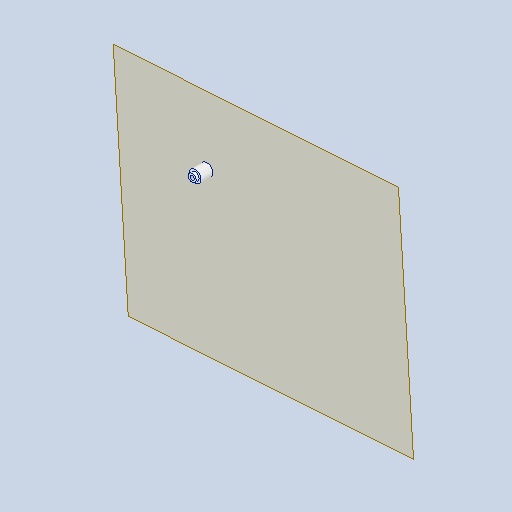
# Autodesk Inventor part: návarek na stěnu
Saved by Autodesk Inventor 2023 (Build 270158000, 158)
## iProperties
Created: 2023-04-03
Part Number: návarek na stěnu
Material: Aluminum 6061
Document SubType Name: Modeling
Designer: lukyv
Density: 2.7 g/cm^3
Appearance: Aluminum - Flat
Mass: 0.445321 g
Surface Area: 2.29336 cm^2
Volume: 0.164934 cm^3
Author: lukyv
Autodesk Inventor part; units mm, degrees
ref_plane "YZ Plane" through (0, 0, 0) normal (1, 0, 0) x (0, 1, 0)
ref_plane "XZ Plane" through (0, 0, 0) normal (0, 1, 0) x (-1, 0, 0)
ref_plane "XY Plane" through (0, 0, 0) normal (0, 0, 1) x (1, 0, 0)
ref_plane "Work Plane1" through (28.3366, -1.7115, 0) normal (0, 0, 1) x (0.9978, 0.066, 0)
sketch "Sketch1" plane through (28.3366, -1.7115, 0) normal (0, 0, 1) x (0.9978, 0.066, 0)
  circle A0 centre (-27.2873, 35.7831) radius 3
  circle A1 centre (-27.2873, 35.7831) radius 1
  circle A2 centre (-27.2873, 35.7831) radius 2
  point P0 (-28.1618, 3.5789)
  dimension "d0" = 6
  dimension "d1" = 2
  dimension "d2" = 4
  constraints: 3 centre point, 2 coincident
  measures "d0" diameter of A0
  measures "d1" diameter of A1
  measures "d2" diameter of A2
extrude "Extrusion1" add sketch "Sketch1" along normal blind 7.5 contours A2
extrude "Extrusion2" add sketch "Sketch1" along normal blind 6 contours A0
thread "Thread1" size "M2x0.4" class "6H" standard "ANSI Metric M Profile" full length
body "Solid1"
